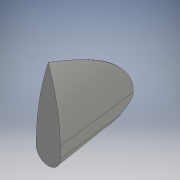
# Autodesk Inventor part: Part2
Saved by Autodesk Inventor 2016 (Build 200138000, 138)
## iProperties
Created: 2016-05-15
Part Number: Part2
Material: Generic
Document SubType Name: Modeling
Designer: Mauricio
Density: 1 g/cm^3
Appearance: Default
Author: Mauricio
Autodesk Inventor part; units mm, degrees
sketch "Sketch4" plane through (0, 0, 0) normal (0, 1, 0) x (-1, 0, 0)
  line L0 (-5800, -1270.1333) -> (-5792.2877, -1270.1333)
  line L1 (-5510.4151, -1125.3409) -> (-5510.4151, -1107.9379)
  line L2 (-5800, -991.6276) -> (-5800, -1125.3409)
  arc A0 (-5800, -1125.3409) -> (-5510.4151, -1125.3409) centre (-5655.2076, -1125.3409) ccw
  arc A1 (-5510.4151, -1125.3409) -> (-5655.2076, -197.2614) centre (-8501.4039, -1116.6394) ccw
  arc A2 (-5655.2076, -197.2614) -> (-5800, -1125.3409) centre (-3181.7697, -1058.4843) ccw
  line L3 (-5792.2877, -1270.1333) -> (-5510.4151, -1270.1333)
  line L4 (-5510.4151, -1270.1333) -> (-5510.4151, -1125.3409)
  line L5 (-5792.2877, -1125.3409) -> (-5792.2877, -1270.1333)
  point P0 (0, 0)
  point P1 (0, 0)
  constraints: 12 end point, 9 point on circle, 3 centre point, 3 tangent, 2 horizontal, 2 parallel, 2 perpendicular
extrude "Extrusion1" add sketch "Sketch4" along normal blind 1000 draft -7 contours A0 L2 A2 A1 L1
ref_plane "Work Plane4" through (5800, 0, -1288.0909) normal (0, 0, 1) x (-0.1218693, 0.9925462, 0)
ref_plane "Work Plane3" through (5800, 0, -1125.3409) normal (0, 0, 1) x (-0.1218693, 0.9925462, 0)
ref_plane "Work Plane5" through (5851, 0, 0) normal (1, 0, 0) x (0, 1, 0)
ref_plane "Work Plane6" through (0, 0, -1300) normal (0, 0, 1) x (1, 0, 0)
sketch "Sketch8" plane through (0, 0, -1300) normal (0, 0, 1) x (1, 0, 0)
  line L0 (5800, 0) -> (5510.4151, 0) projected
  line L1 (5655.2076, 0) -> (5655.2076, 1007.4423)
  line L2 (5800, 0) -> (5510.4151, 0)
  ellipse E0 centre (5655.2076, 0) end of major axis (5655.2076, 1007.4423) minor radius 144.7924 (5800, 0) -> (5510.4151, 0) ccw
  point P0 (0, 0)
  constraints: 4 end point, 1 coincident, 1 collinear, 1 horizontal, 1 midpoint, 1 vertical, 5 other
extrude "Extrusion4" cut sketch "Sketch8" along normal blind 1274.25 keep common part
ref_plane "Work Plane7" through (5882, 0, 0) normal (1, 0, 0) x (0, 1, 0)
sketch "Sketch9" plane through (5882, 0, 0) normal (1, 0, 0) x (0, 1, 0)
  line L0 (0, -1107.9379) -> (0, -197.2614) projected
  line L1 (0, -197.2614) -> (0, -989.8992)
  line L2 (0, -1270.1333) -> (0, -1125.3409) projected
  line L3 (0, -1270.1333) -> (0, -989.8992)
  line L4 (1000, -741.3614) -> (1000, -1108.1184) projected
  line L5 (1000, -989.8992) -> (1000, -567.7514) construction
  line L6 (1000, -567.7514) -> (0, -197.2614) construction
  spline S0 degree 2 poles (1000, -989.8992) (1000, -567.7514) (0, -197.2614) knots 1 1 1 2 2 2
  line L7 (1000, -989.8992) -> (1000, -1167.4476) construction
  line L8 (1000, -1125.3409) -> (1000, -1147.3488) projected
  line L9 (1000, -1167.4476) -> (0, -1270.1333) construction
  spline S1 degree 2 poles (1000, -989.8992) (1000, -1167.4476) (0, -1270.1333) knots 1 1 1 2 2 2
  point P0 (0, 0)
  constraints: 4 end point, 3 collinear, 2 point on line, 6 other
extrude "Extrusion5" cut sketch "Sketch9" against normal blind 1274.25 keep common part
body "Solid1"
